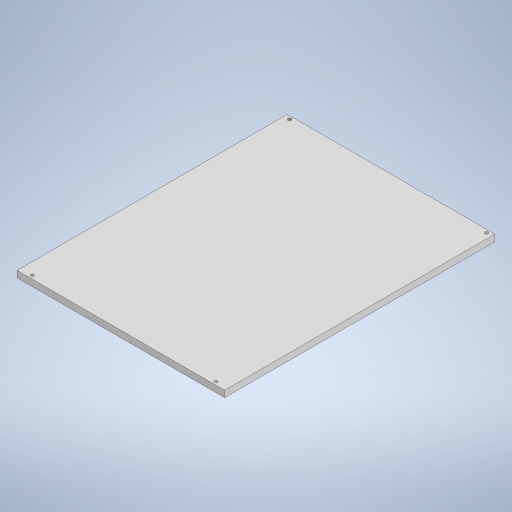
# Autodesk Inventor part: дно_пробитое
Saved by Autodesk Inventor 2024.2 (Build 282272000, 272)
## iProperties
Created: 2025-11-21
Part Number: дно_пробитое
Material: Типовые
Document SubType Name: Modeling
Designer: Zakhar
Density: 1 g/cm^3
Appearance: По умолчанию
Author: Zakhar
Autodesk Inventor part; units mm, degrees
ref_plane "YZ Plane" through (0, 0, 0) normal (1, 0, 0) x (0, 1, 0)
ref_plane "XZ Plane" through (0, 0, 0) normal (0, 1, 0) x (-1, 0, 0)
ref_plane "XY Plane" through (0, 0, 0) normal (0, 0, 1) x (1, 0, 0)
sketch "Эскиз1" plane through (0, 0, 0) normal (0, 1, 0) x (-1, 0, 0)
  line L0 (0, 250) -> (192, 250)
  line L1 (192, 250) -> (192, 0)
  line L2 (192, 0) -> (0, 0)
  line L3 (0, 0) -> (0, 250)
  circle A0 centre (11, 247) radius 1.5
  circle A1 centre (181, 247) radius 1.5
  circle A2 centre (5, 3) radius 1.5
  circle A3 centre (187, 3) radius 1.5
  line L4 (186, 6) -> (6, 6)
  line L5 (6, 6) -> (6, 244)
  line L6 (6, 244) -> (186, 244)
  line L7 (186, 244) -> (186, 6)
  dimension "d0" = 192
  dimension "d1" = 170
  dimension "d2" = 250
  dimension "d3" = 11
  dimension "d4" = 3
  dimension "d5" = 3
  dimension "d6" = 3
  dimension "d7" = 3
  dimension "d8" = 3
  dimension "d9" = 5
  dimension "d10" = 3
  dimension "d11" = 3
  dimension "d12" = 5
  dimension "d13" = 3
  dimension "d16" = 238
  dimension "d18" = 180
  dimension "d19" = 6
  dimension "d20" = 6
  constraints: 16 end point, 4 centre point, 4 parallel, 2 horizontal, 2 perpendicular, 1 coincident
  measures "d0" distance of L0.start L0.end
  measures "d1" distance of A0.centre A1.centre
  measures "d2" distance of L2.end L0.start
  measures "d3" distance from line of L3 A0.centre
  measures "d4" diameter of A0
  measures "d5" distance from line of L0 A0.centre
  measures "d6" distance from line of L0 A1.centre
  measures "d7" diameter of A1
  measures "d8" diameter of A2
  measures "d9" distance from line of A2.centre L3
  measures "d10" distance from line of L2 A2.centre
  measures "d11" diameter of A3
  measures "d12" distance from line of L1 A3.centre
  measures "d13" distance from line of L2 A3.centre
  measures "d16" distance of L4.end L5.end
  measures "d18" distance of L4.start L4.end
  measures "d19" distance between parallel lines of L2 L4
  measures "d20" distance between parallel lines of L3 L5
extrude "Выдавливание1" add sketch "Эскиз1" along normal blind 6 contours L0 L1 L2 L3 | L4 L5 L6 L7
